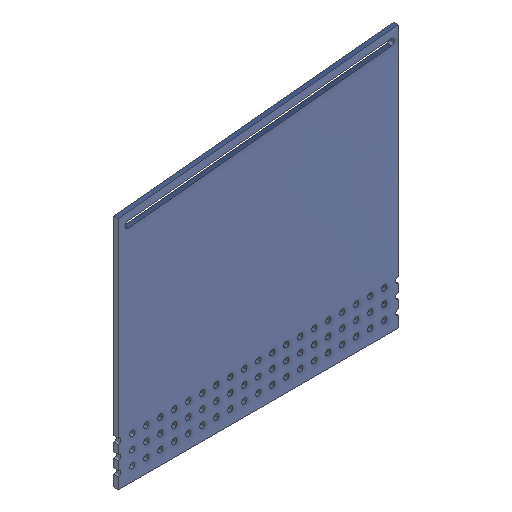
# Autodesk Inventor part: Guia - Intake
Saved by Autodesk Inventor 2025.3 (Build 293356000, 356)
## iProperties
Created: 2026-05-13
Part Number: Guia - Intake
Material: Genérico
Document SubType Name: Modeling
Designer: djair.oliveira
Density: 1 g/cm^3
Appearance: Padrão
Author: djair.oliveira
Autodesk Inventor part; units mm, degrees
ref_plane "YZ Plane" through (0, 0, 0) normal (1, 0, 0) x (0, 1, 0)
ref_plane "XZ Plane" through (0, 0, 0) normal (0, 1, 0) x (-1, 0, 0)
ref_plane "XY Plane" through (0, 0, 0) normal (0, 0, 1) x (1, 0, 0)
sketch "Esboço1" plane through (0, 0, 0) normal (1, 0, 0) x (0, 1, 0)
  line L0 (0, 0) -> (203.2, 0)
  line L1 (203.2, 0) -> (228.6, -254)
  line L2 (228.6, -254) -> (0, -254)
  line L3 (0, -254) -> (0, 0)
  circle A0 centre (12.7, 0) radius 2.5
  circle A1 centre (25.4, 0) radius 2.5
  circle A2 centre (38.1, 0) radius 2.5
  circle A3 centre (38.1, -12.7) radius 2.5
  circle A4 centre (25.4, -12.7) radius 2.5
  circle A5 centre (12.7, -12.7) radius 2.5
  circle A6 centre (38.1, -25.4) radius 2.5
  circle A7 centre (25.4, -25.4) radius 2.5
  circle A8 centre (12.7, -25.4) radius 2.5
  circle A9 centre (38.1, -38.1) radius 2.5
  circle A10 centre (25.4, -38.1) radius 2.5
  circle A11 centre (12.7, -38.1) radius 2.5
  circle A12 centre (38.1, -50.8) radius 2.5
  circle A13 centre (25.4, -50.8) radius 2.5
  circle A14 centre (12.7, -50.8) radius 2.5
  circle A15 centre (38.1, -63.5) radius 2.5
  circle A16 centre (25.4, -63.5) radius 2.5
  circle A17 centre (12.7, -63.5) radius 2.5
  circle A18 centre (38.1, -76.2) radius 2.5
  circle A19 centre (25.4, -76.2) radius 2.5
  circle A20 centre (12.7, -76.2) radius 2.5
  circle A21 centre (38.1, -88.9) radius 2.5
  circle A22 centre (25.4, -88.9) radius 2.5
  circle A23 centre (12.7, -88.9) radius 2.5
  circle A24 centre (38.1, -101.6) radius 2.5
  circle A25 centre (25.4, -101.6) radius 2.5
  circle A26 centre (12.7, -101.6) radius 2.5
  circle A27 centre (38.1, -114.3) radius 2.5
  circle A28 centre (25.4, -114.3) radius 2.5
  circle A29 centre (12.7, -114.3) radius 2.5
  circle A30 centre (38.1, -127) radius 2.5
  circle A31 centre (25.4, -127) radius 2.5
  circle A32 centre (12.7, -127) radius 2.5
  circle A33 centre (38.1, -139.7) radius 2.5
  circle A34 centre (25.4, -139.7) radius 2.5
  circle A35 centre (12.7, -139.7) radius 2.5
  circle A36 centre (38.1, -152.4) radius 2.5
  circle A37 centre (25.4, -152.4) radius 2.5
  circle A38 centre (12.7, -152.4) radius 2.5
  circle A39 centre (38.1, -165.1) radius 2.5
  circle A40 centre (25.4, -165.1) radius 2.5
  circle A41 centre (12.7, -165.1) radius 2.5
  circle A42 centre (38.1, -177.8) radius 2.5
  circle A43 centre (25.4, -177.8) radius 2.5
  circle A44 centre (12.7, -177.8) radius 2.5
  circle A45 centre (38.1, -190.5) radius 2.5
  circle A46 centre (25.4, -190.5) radius 2.5
  circle A47 centre (12.7, -190.5) radius 2.5
  circle A48 centre (38.1, -203.2) radius 2.5
  circle A49 centre (25.4, -203.2) radius 2.5
  circle A50 centre (12.7, -203.2) radius 2.5
  circle A51 centre (38.1, -215.9) radius 2.5
  circle A52 centre (25.4, -215.9) radius 2.5
  circle A53 centre (12.7, -215.9) radius 2.5
  circle A54 centre (38.1, -228.6) radius 2.5
  circle A55 centre (25.4, -228.6) radius 2.5
  circle A56 centre (12.7, -228.6) radius 2.5
  circle A57 centre (38.1, -241.3) radius 2.5
  circle A58 centre (25.4, -241.3) radius 2.5
  circle A59 centre (12.7, -241.3) radius 2.5
  circle A60 centre (38.1, -254) radius 2.5
  circle A61 centre (25.4, -254) radius 2.5
  circle A62 centre (12.7, -254) radius 2.5
  circle A63 centre (203.4985, -2.9851) radius 3
  circle A64 centre (204.0955, -8.9553) radius 3
  circle A65 centre (204.6926, -14.9256) radius 3
  circle A66 centre (205.2896, -20.8958) radius 3
  circle A67 centre (205.8866, -26.866) radius 3
  circle A68 centre (206.4836, -32.8362) radius 3
  circle A69 centre (207.0806, -38.8065) radius 3
  circle A70 centre (207.6777, -44.7767) radius 3
  circle A71 centre (208.2747, -50.7469) radius 3
  circle A72 centre (208.8717, -56.7171) radius 3
  circle A73 centre (209.4687, -62.6873) radius 3
  circle A74 centre (210.0658, -68.6576) radius 3
  circle A75 centre (210.6628, -74.6278) radius 3
  circle A76 centre (211.2598, -80.598) radius 3
  circle A77 centre (211.8568, -86.5682) radius 3
  circle A78 centre (212.4538, -92.5385) radius 3
  circle A79 centre (213.0509, -98.5087) radius 3
  circle A80 centre (213.6479, -104.4789) radius 3
  circle A81 centre (214.2449, -110.4491) radius 3
  circle A82 centre (214.8419, -116.4194) radius 3
  circle A83 centre (215.439, -122.3896) radius 3
  circle A84 centre (216.036, -128.3598) radius 3
  circle A85 centre (216.633, -134.33) radius 3
  circle A86 centre (217.23, -140.3002) radius 3
  circle A87 centre (217.827, -146.2705) radius 3
  circle A88 centre (218.4241, -152.2407) radius 3
  circle A89 centre (219.0211, -158.2109) radius 3
  circle A90 centre (219.6181, -164.1811) radius 3
  circle A91 centre (220.2151, -170.1514) radius 3
  circle A92 centre (220.8122, -176.1216) radius 3
  circle A93 centre (221.4092, -182.0918) radius 3
  circle A94 centre (222.0062, -188.062) radius 3
  circle A95 centre (222.6032, -194.0323) radius 3
  circle A96 centre (223.2002, -200.0025) radius 3
  circle A97 centre (223.7973, -205.9727) radius 3
  circle A98 centre (224.3943, -211.9429) radius 3
  circle A99 centre (224.9913, -217.9131) radius 3
  circle A100 centre (225.5883, -223.8834) radius 3
  circle A101 centre (226.1854, -229.8536) radius 3
  circle A102 centre (226.7824, -235.8238) radius 3
  circle A103 centre (227.3794, -241.794) radius 3
  circle A104 centre (227.9764, -247.7643) radius 3
  circle A105 centre (228.5734, -253.7345) radius 3
  line L4 (203.2, 0) -> (213.2499, 0)
  line L5 (213.2499, 0) -> (238.6499, -254)
  line L6 (238.6499, -254) -> (228.6, -254)
  line L7 (227.9764, -247.7643) -> (204.0955, -8.9553) construction
  line L8 (230.9615, -247.4657) -> (207.0806, -8.6568)
  line L9 (201.1104, -9.2538) -> (224.9913, -248.0628)
  arc A106 (224.9913, -248.0628) -> (230.9615, -247.4657) centre (227.9764, -247.7643) ccw
  arc A107 (207.0806, -8.6568) -> (201.1104, -9.2538) centre (204.0955, -8.9553) ccw
  point P0 (40.6, 0)
  point P1 (35.6, 0)
  point P2 (27.9, 0)
  point P3 (22.9, 0)
  point P4 (15.2, 0)
  point P5 (10.2, 0)
  point P6 (10.2, -254)
  point P7 (15.2, -254)
  point P8 (22.9, -254)
  point P9 (27.9, -254)
  point P10 (35.6, -254)
  point P11 (40.6, -254)
  point P12 (203.797, -5.9702)
  point P13 (204.394, -11.9404)
  point P14 (204.9911, -17.9107)
  point P15 (205.5881, -23.8809)
  point P16 (206.1851, -29.8511)
  point P17 (206.7821, -35.8213)
  point P18 (207.3792, -41.7916)
  point P19 (207.9762, -47.7618)
  point P20 (208.5732, -53.732)
  point P21 (209.1702, -59.7022)
  point P22 (209.7672, -65.6725)
  point P23 (210.3643, -71.6427)
  point P24 (210.9613, -77.6129)
  point P25 (211.5583, -83.5831)
  point P26 (212.1553, -89.5533)
  point P27 (212.7524, -95.5236)
  point P28 (213.3494, -101.4938)
  point P29 (213.9464, -107.464)
  point P30 (214.5434, -113.4342)
  point P31 (215.1404, -119.4045)
  point P32 (215.7375, -125.3747)
  point P33 (216.3345, -131.3449)
  point P34 (216.9315, -137.3151)
  point P35 (217.5285, -143.2854)
  point P36 (218.1256, -149.2556)
  point P37 (218.7226, -155.2258)
  point P38 (219.3196, -161.196)
  point P39 (219.9166, -167.1662)
  point P40 (220.5136, -173.1365)
  point P41 (221.1107, -179.1067)
  point P42 (221.7077, -185.0769)
  point P43 (222.3047, -191.0471)
  point P44 (222.9017, -197.0174)
  point P45 (223.4988, -202.9876)
  point P46 (224.0958, -208.9578)
  point P47 (224.6928, -214.928)
  point P48 (225.2898, -220.8983)
  point P49 (225.8868, -226.8685)
  point P50 (226.4839, -232.8387)
  point P51 (227.0809, -238.8089)
  point P52 (227.6779, -244.7791)
  point P53 (228.2749, -250.7494)
  point P54 (228.2749, -250.7494)
  point P55 (227.6779, -244.7791)
  point P56 (227.0809, -238.8089)
  point P57 (226.4839, -232.8387)
  point P58 (225.8868, -226.8685)
  point P59 (225.2898, -220.8983)
  point P60 (224.6928, -214.928)
  point P61 (224.0958, -208.9578)
  point P62 (223.4988, -202.9876)
  point P63 (222.9017, -197.0174)
  point P64 (222.3047, -191.0471)
  point P65 (221.7077, -185.0769)
  point P66 (221.1107, -179.1067)
  point P67 (220.5136, -173.1365)
  point P68 (219.9166, -167.1662)
  point P69 (219.3196, -161.196)
  point P70 (218.7226, -155.2258)
  point P71 (218.1256, -149.2556)
  point P72 (217.5285, -143.2854)
  point P73 (216.9315, -137.3151)
  point P74 (216.3345, -131.3449)
  point P75 (215.7375, -125.3747)
  point P76 (215.1404, -119.4045)
  point P77 (214.5434, -113.4342)
  point P78 (213.9464, -107.464)
  point P79 (213.3494, -101.4938)
  point P80 (212.7524, -95.5236)
  point P81 (212.1553, -89.5533)
  point P82 (211.5583, -83.5831)
  point P83 (210.9613, -77.6129)
  point P84 (210.3643, -71.6427)
  point P85 (209.7672, -65.6725)
  point P86 (209.1702, -59.7022)
  point P87 (208.5732, -53.732)
  point P88 (207.9762, -47.7618)
  point P89 (207.3792, -41.7916)
  point P90 (206.7821, -35.8213)
  point P91 (206.1851, -29.8511)
  point P92 (205.5881, -23.8809)
  point P93 (204.9911, -17.9107)
  point P94 (204.394, -11.9404)
  point P95 (203.797, -5.9702)
  point P96 (216.036, -128.3598)
  point P97 (207.0806, -8.6568)
  point P98 (224.9913, -248.0628)
  point P99 (201.1104, -9.2538)
  dimension "d16" = 6
  dimension "d0" = 254
  dimension "d1" = 228.6
  dimension "d2" = 203.2
  dimension "d3" = 5
  dimension "d4" = 12.7
  dimension "d5" = 12.7
  dimension "d6" = 12.7
  dimension "d9" = 12.7
  dimension "d19" = 6
  dimension "d26" = 252
  dimension "d27" = 10
  constraints: 65 centre point, 20 end point, 4 point on circle, 4 tangent, 3 point on line, 2 equal radius, 2 horizontal, 2 parallel, 1 collinear, 1 midpoint, 1 perpendicular, 1 vertical, 340 other
  measures "d0" distance of L2.end L0.start
  measures "d1" distance of L2.start L2.end
  measures "d2" distance of L0.start L0.end
  measures "d3" diameter of A2
  measures "d4" distance of A1.centre A2.centre
  measures "d5" distance of A1.centre A0.centre
  measures "d6" distance from line of L3 A0.centre
  measures "d9" distance of A2.centre A3.centre
  measures "d19" distance of point (203.499, -2.985) L7.end
  measures "d26" distance of point (228.573, -253.734) point (203.499, -2.985)
  measures "d27" distance from line of point (228.275, -250.749) L5
extrude "Extrusão1" add sketch "Esboço1" along normal blind 4 contours L0 A63 A64 L9 A104 A105 L2 A60 A61 A62 L3 A0 A1 A2 | L4 A63 L1 | L1 A63 | A63 L4 L5 L6 A105 A104 L8 A64 | L6 L1 A105 | A105 L1 L2
equation "\"d5\" = d4"
